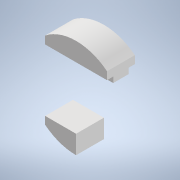
# Autodesk Inventor part: uchwyt_silników
Saved by Autodesk Inventor 2022 (Build 260153000, 153)
## iProperties
Created: 2022-12-24
Part Number: uchwyt_silników
Material: Generic
Document SubType Name: Modeling
Designer: Kamil
Density: 1 g/cm^3
Appearance: Default
Author: Kamil
Autodesk Inventor part; units mm, degrees
ref_plane "YZ Plane" through (0, 0, 0) normal (1, 0, 0) x (0, 1, 0)
ref_plane "XZ Plane" through (0, 0, 0) normal (0, 1, 0) x (-1, 0, 0)
sketch "Sketch1" plane through (0, 0, 0) normal (0, 0, 1) x (1, 0, 0)
  line L0 (6, 4) -> (6, 1) projected
  arc A0 (6, 4) -> (5, 5) centre (5, 4) ccw projected
  line L1 (-5, 5) -> (5, 5) projected
  arc A1 (-5, 5) -> (-6, 4) centre (-5, 4) ccw projected
  line L2 (-6, -4) -> (-6, 4) projected
  arc A2 (-6, -4) -> (-5, -5) centre (-5, -4) ccw projected
  line L3 (0, -5) -> (-5, -5) projected
  arc A3 (0, -5) -> (1, -4) centre (0, -4) ccw projected
  line L4 (1, -1) -> (1, -4) projected
  arc A4 (2, 0) -> (1, -1) centre (2, -1) ccw projected
  line L5 (5, 0) -> (2, 0) projected
  arc A5 (5, 0) -> (6, 1) centre (5, 1) ccw projected
  circle A6 centre (0, 0) radius 0.5 projected
  circle A7 centre (3.5, 2.5) radius 1.5 projected
  circle A8 centre (-3.5, -2.5) radius 1.5 projected
  circle A9 centre (-3, 3) radius 0.5 projected
  circle A10 centre (0, 0) radius 9.5 projected
  line L6 (0, 9.5) -> (0, 8)
  circle A11 centre (0, 0) radius 8
  line L7 (-5, 5) -> (-5, 6.245)
  line L8 (5, 5) -> (5, 6.245)
  line L9 (-5, -5) -> (-5, -6.245)
  line L10 (0, -5) -> (0, -8)
  point P0 (0, 0)
  dimension "d0" = 1.5
  constraints: 10 end point, 6 point on circle, 2 parallel, 2 vertical, 1 centre point, 1 coincident, 1 perpendicular, 1 vertical alignment, 1 other
  measures "d0" distance of L6.start L6.end
ref_plane "Work Plane1" through (-6, -5, -4.5) normal (0, 0, -1) x (0, 1, 0)
extrude "Extrusion1" add sketch "Sketch1" against normal up to surface (4.5 mm away) contours L1 L7 A11 L8 | L9 L3 L10 A11
sketch "Sketch2" plane through (-5, 5, 0) normal (0, -1, 0) x (1, 0, 0)
  line L0 (0, -1) -> (10, -1) projected
  line L1 (0, -3.5) -> (10, -3.5) projected
  line L2 (10, -1) -> (10, -3.5)
  line L3 (0, -1) -> (0, -3.5)
  line L4 (0, 0) -> (0, -4.5) projected
  point P0 (5, 0)
  constraints: 4 end point, 1 collinear, 1 perpendicular
extrude "Extrusion2" add sketch "Sketch2" along normal blind 0.9
sketch "Sketch3" plane through (5, 5, 0) normal (1, 0, 0) x (0, 0, -1)
  line L0 (4.5, 0) -> (4.5, 1.245) projected
  line L1 (0, 1.245) -> (4.5, 1.245) projected
  line L2 (0, 0) -> (0, 1.245) projected
  line L3 (0, 0) -> (1, 0) projected
  line L4 (1, 0) -> (1, -0.9) projected
  line L5 (3.5, -0.9) -> (1, -0.9) projected
  line L6 (3.5, 0) -> (3.5, -0.9) projected
  line L7 (3.5, 0) -> (4.5, 0) projected
  line L8 (1, -0.9) -> (3.5, -0.9) projected
  line L9 (1, -0.9) -> (1.1961, -0.9)
  line L10 (1.1961, -0.9) -> (1.1961, 0)
  line L11 (1.1961, 0) -> (1, 0)
  line L12 (1, 0) -> (1, -0.9)
  point P0 (0, -5)
  constraints: 8 end point, 2 parallel, 1 horizontal, 1 perpendicular
extrude "Extrusion3" cut sketch "Sketch3" against normal through all contours L5 L4 L11 L10
sketch "Sketch4" plane through (0, -8, 0) normal (1, 0, 0) x (0, 0, -1)
  line L0 (4.5, 0) -> (4.5, 3) projected
  line L1 (0, 3) -> (4.5, 3) projected
  line L2 (0, 0) -> (0, 3) projected
  line L3 (0, 0) -> (4.5, 0) projected
  point P0 (0, 8)
extrude "Extrusion4" cut sketch "Sketch4" against normal through all
ref_plane "Work Plane2" through (0, -0.2011, -23) normal (0, 0, 1) x (1, 0, 0)
mirror "Mirror1" about plane through (0, -0.2011, -23) normal (0, 0, 1)
sketch "Sketch5" plane through (0, 0, -4.5) normal (0, 0, -1) x (-1, 0, 0)
  arc A0 (5, 6.245) -> (-5, 6.245) centre (0, 0) ccw projected
  line L0 (-5, 5) -> (-5, 6.245) projected
  line L1 (5, 5) -> (-5, 5) projected
  line L2 (5, 6.245) -> (5, 5) projected
  line L3 (-1.7, 5) -> (-2.3, 5) projected
  line L4 (4.1641, 5) -> (-4.1641, 5) projected
  point P0 (0, 0)
extrude "Extrusion5" add sketch "Sketch5" along normal blind 6
mirror "Mirror2" about plane through (0, -0.2011, -23) normal (0, 0, 1)
sketch "Sketch6" plane through (0, 0, -10.5) normal (0, 0, -1) x (-1, 0, 0)
  arc A0 (-4.3225, 4.9221) -> (-5.9696, 0.6989) centre (2.06, 0) ccw projected
  line L0 (-4.065, 4.6) -> (4.065, 4.6) projected
  arc A1 (4.065, -4.6) -> (4.065, 4.6) centre (-2.06, 0) ccw projected
  line L1 (4.065, -4.6) -> (-4.065, -4.6) projected
  arc A2 (-4.065, 4.6) -> (-4.065, -4.6) centre (2.06, 0) ccw projected
  circle A3 centre (0, 0) radius 1 projected
  arc A4 (4.3225, -4.9221) -> (4.3225, 4.9221) centre (-2.06, 0) ccw projected
  arc A5 (-4.3225, 4.9221) -> (-4.3225, -4.9221) centre (2.06, 0) ccw projected
  arc A6 (-4.065, 4.6) -> (-4.065, -4.6) centre (2.06, 0) ccw projected
  arc A7 (-4.3225, 4.9221) -> (-4.3225, -4.9221) centre (2.06, 0) ccw projected
  line L2 (1, -5) -> (4.1641, -5) projected
  line L3 (-1, -5) -> (1, -5) projected
  line L4 (-1, -5) -> (-4.1641, -5) projected
  line L5 (0, -5) -> (0, -9)
  arc A8 (4.9221, 7.5348) -> (0, -9) centre (0, 0) ccw
  line L6 (0, -9) -> (16.2029, -9)
  line L7 (4.1641, -5) -> (16.2029, -5)
  line L8 (16.2029, -5) -> (16.2029, -9)
  arc A9 (-1.0781, -8) -> (-0.796, -7.9603) centre (-2.06, 0) ccw
  arc A10 (5, 6.245) -> (-5, 6.245) centre (0, 0) ccw projected
  line L9 (-5, 6.245) -> (-5, 5) projected
  line L10 (-5, 5) -> (5, 5) projected
  line L11 (5, 5) -> (5, 6.245) projected
  line L12 (-9, 0) -> (-9, 10.5642)
  arc A11 (5, 6.245) -> (-5, 6.245) centre (0, 0) ccw projected
  line L13 (0, 8) -> (-9, 8)
  line L14 (6, 0) -> (8, 0)
  line L15 (8, 0) -> (8, -5)
  line L16 (8, -5) -> (8, -3.5)
  line L17 (8, -3.5) -> (5.2004, -3.5)
  circle A12 centre (0, 0) radius 8
  circle A13 centre (0, 0) radius 9
  line L18 (-4.1641, -5) -> (-4.349, -5)
  line L19 (4.3225, -4.9221) -> (4.2617, -5)
  line L20 (-4.3225, -4.9221) -> (-4.2566, -5)
  line L21 (-4.3225, 4.9221) -> (-4.2566, 5)
  line L22 (-5, 5) -> (5, 5) projected
  line L23 (4.3225, 4.9221) -> (4.2617, 5)
  point P0 (0, 0)
  point P1 (-4.2566, 5)
  point P2 (4.2617, 5)
  point P3 (5, 6.245)
  dimension "d11" = 4
  dimension "d12" = 2
  dimension "d13" = 1.5
  constraints: 30 end point, 9 point on circle, 6 point on line, 4 horizontal, 4 perpendicular, 3 coincident, 3 tangent, 2 centre point, 2 midpoint, 2 vertical, 6 other
  measures "d11" distance of L5.start L5.end
  measures "d12" distance of L14.start L14.end
  measures "d13" distance of L15.end L16.end
extrude "Extrusion6" add sketch "Sketch6" along normal blind 6 contours A0 A5 L20 L18 L4 L3 L5 A12 L9 L10 L21 | L10 L9 A10 L11 | L10 L11 A12 L14 A4 L23 | A12 L5 A8 L13 A10 | L14 A12 L17 A4 | A8 L12 L13 | A12 L7 A13 L5 | L5 L3 L2 L7 A12 | L15 L17 A12 | A13 L7 L8 L6
sketch "Sketch7" plane through (0, 0, -10.5) normal (0, 0, 1) x (1, 0, 0)
  arc A0 (5, 6.245) -> (0, 8) centre (0, 0) ccw projected
  line L0 (5, 6.245) -> (5, 5) projected
  line L1 (5, 5) -> (4.2566, 5) projected
  line L2 (4.3225, 4.9221) -> (4.2566, 5) projected
  arc A1 (4.3225, -4.9221) -> (4.3225, 4.9221) centre (-2.06, 0) ccw projected
  line L3 (4.2566, -5) -> (4.3225, -4.9221) projected
  line L4 (-16.2029, -5) -> (4.2566, -5) projected
  line L5 (-16.2029, -9) -> (-16.2029, -5) projected
  line L6 (0, -9) -> (-16.2029, -9) projected
  arc A2 (0, -9) -> (9, 0) centre (0, 0) ccw projected
  line L7 (9, 8) -> (9, 0) projected
  line L8 (0, 8) -> (9, 8) projected
  line L9 (-5, 5) -> (-5, 6.245) projected
  arc A3 (-5, 6.245) -> (-8, 0) centre (0, 0) ccw projected
  line L10 (-8, -3.5) -> (-8, 0) projected
  line L11 (-5.2004, -3.5) -> (-8, -3.5) projected
  arc A4 (-4.3225, 4.9221) -> (-5.2004, -3.5) centre (2.06, 0) ccw projected
  line L12 (-4.2617, 5) -> (-4.3225, 4.9221) projected
  line L13 (-4.2617, 5) -> (-5, 5) projected
  line L14 (-16.2029, -9) -> (9, -9)
  line L15 (9, -9) -> (9, 8)
  line L16 (9, 8) -> (-16.2029, 8)
  line L17 (-16.2029, 8) -> (-16.2029, -9)
  point P0 (0, 0)
  point P1 (9, 0)
  constraints: 8 end point, 2 parallel, 1 horizontal, 1 perpendicular
extrude "Extrusion7" add sketch "Sketch7" against normal blind 6 contours L15 L14 A2
sketch "Sketch8" plane through (0, 0, -10.5) normal (0, 0, 1) x (1, 0, 0)
  line L0 (-5, 5) -> (-5, 6.245) projected
  arc A0 (-5, 6.245) -> (-8, 0) centre (0, 0) ccw projected
  line L1 (-8, -3.5) -> (-8, 0) projected
  line L2 (-5.2004, -3.5) -> (-8, -3.5) projected
  arc A1 (-4.3225, 4.9221) -> (-5.2004, -3.5) centre (2.06, 0) ccw projected
  line L3 (-4.2617, 5) -> (-4.3225, 4.9221) projected
  line L4 (-4.2617, 5) -> (-5, 5) projected
  arc A2 (5, 6.245) -> (0, 8) centre (0, 0) ccw projected
  line L5 (5, 6.245) -> (5, 5) projected
  line L6 (5, 5) -> (4.2566, 5) projected
  line L7 (4.3225, 4.9221) -> (4.2566, 5) projected
  arc A3 (4.3225, -4.9221) -> (4.3225, 4.9221) centre (-2.06, 0) ccw projected
  line L8 (4.2566, -5) -> (4.3225, -4.9221) projected
  line L9 (-16.2029, -5) -> (4.2566, -5) projected
  line L10 (-16.2029, -9) -> (-16.2029, -5) projected
  line L11 (-16.2029, -9) -> (9, -9) projected
  line L12 (9, 8) -> (9, -9) projected
  line L13 (0, 8) -> (9, 8) projected
  point P0 (0, 0)
extrude "Extrusion8" add sketch "Sketch8" along normal blind 3
sketch "Sketch9" plane through (0, 0, -16.5) normal (0, 0, -1) x (-1, 0, 0)
  line L0 (16.2029, -5) -> (-4.2566, -5) projected
  line L1 (-4.2566, -5) -> (-4.3225, -4.9221) projected
  arc A0 (-4.3225, 4.9221) -> (-4.3225, -4.9221) centre (2.06, 0) ccw projected
  line L2 (-4.3225, 4.9221) -> (-4.2566, 5) projected
  line L3 (-4.2566, 5) -> (4.2617, 5) projected
  line L4 (4.2617, 5) -> (4.3225, 4.9221) projected
  arc A1 (5.2004, -3.5) -> (4.3225, 4.9221) centre (-2.06, 0) ccw projected
  line L5 (5.2004, -3.5) -> (8, -3.5) projected
  line L6 (8, -3.5) -> (8, 0) projected
  arc A2 (8, 0) -> (0, 8) centre (0, 0) ccw projected
  line L7 (0, 8) -> (-9, 8) projected
  line L8 (-9, 8) -> (-9, -9) projected
  line L9 (-9, -9) -> (16.2029, -9) projected
  line L10 (16.2029, -9) -> (16.2029, -5) projected
  point P0 (0, 0)
extrude "Extrusion9" add sketch "Sketch9" along normal up to surface (6.5 mm away)
sketch "Sketch10" plane through (0, 8, -7.5) normal (0, 1, 0) x (1, 0, 0)
  line L0 (9, 0) -> (9, 15.5) projected
  line L1 (0, 15.5) -> (9, 15.5) projected
  line L2 (0, 0) -> (0, 15.5) projected
  line L3 (9, 0) -> (0, 0) projected
  line L4 (0, 0) -> (0, 15.5) projected
  circle A0 centre (0, 15.5) radius 1.6
  point P0 (0, -7.5)
  dimension "d22" = 3.2
  constraints: 1 centre point, 1 coincident
  measures "d22" diameter of A0
extrude "Extrusion10" cut sketch "Sketch10" against normal blind 3 contours A0 L2 L1 | L1 L2 A0
sketch "Sketch11" plane through (-8, -3.5, -7.5) normal (-1, 0, 0) x (0, 0, 1)
  line L0 (0, 3.5) -> (-15.5, 3.5) projected
  line L1 (-15.5, 0) -> (-15.5, 3.5) projected
  line L2 (0, 0) -> (-15.5, 0) projected
  line L3 (0, 3.5) -> (0, 0) projected
  point P0 (7.5, 3.5)
extrude "Extrusion11" add sketch "Sketch11" along normal up to surface (8.2029 mm away)
sketch "Sketch12" plane through (-16.2029, 0, -7.5) normal (0, 1, 0) x (1, 0, 0)
  line L0 (0, 15.5) -> (0, 0) projected
  line L1 (8.2029, 0) -> (0, 0) projected
  line L2 (8.2029, 0) -> (8.2029, 15.5) projected
  line L3 (8.2029, 15.5) -> (0, 15.5) projected
  line L4 (0, 0) -> (0, 15.5) projected
  line L5 (0, 7.75) -> (8.2029, 7.75)
  line L6 (20.4595, 0) -> (0, 0) projected
  line L7 (0, 7.75) -> (0, 0)
  line L8 (0, 3.875) -> (8.2029, 0)
  line L9 (8.2029, 7.75) -> (7.2029, 7.75)
  line L10 (7.2029, 7.75) -> (0.8029, 7.75)
  line L11 (7.2029, 5.9025) -> (4.0029, 4.055)
  line L12 (4.0029, 4.055) -> (0.8029, 5.9025)
  line L13 (0.8029, 5.9025) -> (0.8029, 9.5975)
  line L14 (0.8029, 9.5975) -> (4.0029, 11.445)
  line L15 (4.0029, 11.445) -> (7.2029, 9.5975)
  line L16 (7.2029, 9.5975) -> (7.2029, 5.9025)
  circle A0 centre (4.0029, 7.75) radius 1.6
  point P0 (16.2029, -7.5)
  dimension "d27" = 1
  dimension "d28" = 6.4
  dimension "d29" = 3.2
  constraints: 22 end point, 5 midpoint, 2 point on line, 1 centre point, 1 coincident, 1 vertical, 13 other
  measures "d27" distance of L5.end L9.end
  measures "d28" distance of L9.end L10.end
  measures "d29" diameter of A0
extrude "Extrusion12" cut sketch "Sketch12" against normal blind 2 contours L13 L14 L15 L16 L5 A0 | L5 A0 L16 L11 L12 L13
extrude "Extrusion13" cut sketch "Sketch12" against normal through all contours A0 L5 | L5 A0
sketch "Sketch13" plane through (-16.2029, 0, -7.5) normal (0, 1, 0) x (1, 0, 0)
  line L0 (0, 15.5) -> (0, 0) projected
  line L1 (8.2029, 0) -> (0, 0) projected
  line L2 (8.2029, 0) -> (8.2029, 15.5) projected
  line L3 (8.2029, 15.5) -> (0, 15.5) projected
  line L4 (7.2029, 5.9025) -> (4.0029, 4.055) projected
  line L5 (4.0029, 4.055) -> (0.8029, 5.9025) projected
  line L6 (0.8029, 5.9025) -> (0.8029, 9.5975) projected
  line L7 (0.8029, 9.5975) -> (4.0029, 11.445) projected
  line L8 (4.0029, 11.445) -> (7.2029, 9.5975) projected
  line L9 (7.2029, 9.5975) -> (7.2029, 5.9025) projected
  circle A0 centre (4.0029, 7.75) radius 1.6 projected
  circle A1 centre (4.0029, 7.75) radius 4.2
  line L10 (8.2029, 0) -> (1.7099, 4.2312)
  point P0 (16.2029, -7.5)
  point P1 (0, 6.4785)
  constraints: 2 end point, 1 coincident, 1 vertical, 4 other
extrude "Extrusion14" cut sketch "Sketch13" against normal up to surface (5 mm away) contours A1 L10 L1 L0
sketch "Sketch14" plane through (-16.2029, -9, -7.5) normal (0, -1, 0) x (1, 0, 0)
  circle A0 centre (4.0029, -7.75) radius 1.6 projected
  line L0 (0, 0) -> (0, -15.5) projected
  line L1 (25.2029, -15.5) -> (0, -15.5) projected
  line L2 (25.2029, -15.5) -> (25.2029, 0) projected
  line L3 (0, 0) -> (25.2029, 0) projected
  line L4 (21.2029, 4) -> (21.2029, 0) projected
  line L5 (11.2029, 4) -> (11.2029, 0) projected
  line L6 (20.4595, 0) -> (21.2029, 0) projected
  line L7 (21.2029, 0) -> (11.2029, 0)
  line L8 (20.4595, 0) -> (0, 0) projected
  line L9 (16.2029, 0) -> (16.2029, -13.9) projected
  line L10 (16.2029, 0) -> (16.2029, -15.5)
  line L11 (4.0029, -7.75) -> (25.2029, -7.75)
  line L12 (25.2029, -15.5) -> (25.2029, 0) projected
  circle A1 centre (16.2029, -7.75) radius 1.5
  point P0 (16.2029, 7.5)
  dimension "d36" = 3
  constraints: 6 end point, 2 collinear, 2 midpoint, 2 point on line, 1 centre point
  measures "d36" diameter of A1
extrude "Extrusion15" cut sketch "Sketch14" against normal blind 5 contours A1 L11 L9 | L9 L11 A1 | A1 L11 L9 | L9 L11 A1
sketch "Sketch15" plane through (-16.2029, -3.5, -23) normal (-1, 0, 0) x (0, 0, 1)
  line L0 (9.0215, 0) -> (9.0215, 3.5) projected
  line L1 (0, 3.5) -> (9.0215, 3.5) projected
  line L2 (0, 0) -> (0, 3.5) projected
  line L3 (9.0215, 0) -> (0, 0) projected
  line L4 (2.4, 3.9989) -> (3.5, 3.9989) projected
  arc A0 (2.4, 3.9989) -> (2, 3.5989) centre (2.4, 3.5989) ccw projected
  line L5 (2, 2.9989) -> (2, 3.5989) projected
  arc A1 (2, 2.9989) -> (2.4, 2.5989) centre (2.4, 2.9989) ccw projected
  line L6 (2.4, 2.5989) -> (3.5, 2.5989) projected
  line L7 (3.5, 2.5989) -> (3.5, 3.9989) projected
  circle A2 centre (2.8, 3.3127) radius 0.4 projected
  line L8 (0, 0) -> (0, 8.4221) projected
  circle A3 centre (0, 4.6105) radius 3.5007
  point P0 (23, 3.5)
  point P1 (0, 8.1112)
  point P2 (3.3199, 3.5)
  constraints: 1 centre point, 1 point on line
extrude "Extrusion16" cut sketch "Sketch15" against normal blind 13 contours L1 A2 L5 A0 L4 A3 | L8 A3 L4 A0 L5 L1 | L1 A2 picked at (2.8995, 3.5263)
mirror "Mirror3" about plane through (0, -0.2011, -23) normal (0, 0, 1)
fillet "Fillet1" radius 5 2 edges at (9, -9, -15.25) (9, -9, -30.75)
sketch "Sketch16" plane through (-16.2029, -9, -38.5) normal (0, -1, 0) x (1, 0, 0)
  line L0 (20.2029, 31) -> (20.2029, 0) projected
  line L1 (0, 31) -> (20.2029, 31) projected
  line L2 (0, 31) -> (0, 0) projected
  line L3 (0, 0) -> (20.2029, 0) projected
  circle A0 centre (4.0029, 23.25) radius 1.6 projected
  circle A1 centre (16.2029, 23.25) radius 1.5 projected
  circle A2 centre (16.2029, 7.75) radius 1.5 projected
  circle A3 centre (4.0029, 7.75) radius 1.6 projected
  circle A4 centre (16.2029, 15.5) radius 1.6 projected
  point P0 (16.2029, 38.5)
extrude "Extrusion17" cut sketch "Sketch16" against normal blind 13 contours A4
body "Solid1"
